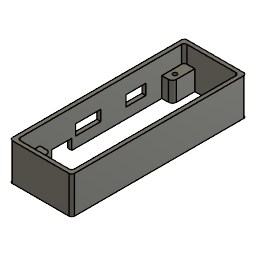
weather_station1 (Autodesk Fusion 360 design; units mm, degrees)
part number: 2026-01-11-18-10-58-376
Autodesk Fusion 360 part; units mm, degrees
sketch "Sketch11" plane through (0, 0, 0) normal (0, 1, 0) x (1, 0, 0)
  line L0 (0, 0) -> (47, 0)
  line L1 (47, 0) -> (47, -132)
  line L2 (47, -132) -> (0, -132)
  line L3 (0, -132) -> (0, 0)
  circle A0 centre (2, -2) radius 2
  circle A1 centre (45, -2) radius 2
  circle A2 centre (45, -130) radius 2
  circle A3 centre (2, -130) radius 2
  line L4 (3, -3) -> (44, -3)
  line L5 (44, -3) -> (44, -129)
  line L6 (44, -129) -> (3, -129)
  line L7 (3, -129) -> (3, -3)
  circle A4 centre (5, -5) radius 2
  circle A5 centre (42, -5) radius 2
  circle A6 centre (42, -127) radius 2
  circle A7 centre (5, -127) radius 2
  line L8 (3, -132) -> (6, -132)
  line L9 (6, -132) -> (6, -121)
  line L10 (6, -121) -> (3, -121)
  line L11 (3, -121) -> (3, -132)
  line L12 (44, -132) -> (41, -132)
  line L13 (41, -132) -> (41, -121)
  line L14 (41, -121) -> (44, -121)
  line L15 (44, -121) -> (44, -132)
  line L16 (3, 0) -> (6, 0)
  line L17 (6, 0) -> (6, -11)
  line L18 (6, -11) -> (3, -11)
  line L19 (3, -11) -> (3, 0)
  line L20 (44, 0) -> (41, 0)
  line L21 (41, 0) -> (41, -11)
  line L22 (41, -11) -> (44, -11)
  line L23 (44, -11) -> (44, 0)
  circle A8 centre (41, -11) radius 1
  circle A9 centre (6, -11) radius 1
  circle A10 centre (41, -121) radius 1
  circle A11 centre (6, -121) radius 1
  line L24 (3, -117) -> (9, -117)
  line L25 (9, -117) -> (9, -129)
  line L26 (9, -129) -> (3, -129)
  line L27 (3, -129) -> (3, -117)
  line L28 (44, -117) -> (38, -117)
  line L29 (38, -117) -> (38, -129)
  line L30 (38, -129) -> (44, -129)
  line L31 (44, -129) -> (44, -117)
  line L32 (44, -15) -> (38, -15)
  line L33 (38, -15) -> (38, -3)
  line L34 (38, -3) -> (44, -3)
  line L35 (44, -3) -> (44, -15)
  line L36 (3, -15) -> (9, -15)
  line L37 (9, -15) -> (9, -3)
  line L38 (9, -3) -> (3, -3)
  line L39 (3, -3) -> (3, -15)
  circle A12 centre (7, -13) radius 2
  circle A13 centre (40, -119) radius 2
  circle A14 centre (7, -119) radius 2
  circle A15 centre (40, -13) radius 2
  dimension "d82" = 47
  dimension "d83" = 132
  constraint horizontal L0
  constraint vertical L1
  constraint horizontal L2
  constraint vertical L3
  constraint coincident L0.start L3.end
  constraint tangent L0 A0
  constraint tangent L0 A1
  constraint tangent L1 A2
  constraint tangent L2 A3
  constraint horizontal L4
  constraint vertical L5
  constraint horizontal L6
  constraint vertical L7
  constraint tangent L4 A4
  constraint tangent L4 A5
  constraint tangent L5 A6
  constraint tangent L6 A7
  constraint horizontal L8
  constraint vertical L9
  constraint horizontal L10
  constraint vertical L11
  constraint coincident L2 L8.start
  constraint horizontal L12
  constraint vertical L13
  constraint horizontal L14
  constraint vertical L15
  constraint coincident L2 L12.start
  constraint horizontal L16
  constraint vertical L17
  constraint horizontal L18
  constraint vertical L19
  constraint coincident L0 L16.start
  constraint horizontal L20
  constraint vertical L21
  constraint horizontal L22
  constraint vertical L23
  constraint coincident L0 L20.start
  constraint coincident L21.end L22.start
  constraint coincident L17.end L18.start
  constraint coincident L13.end L14.start
  constraint coincident L9.end L10.start
  constraint horizontal L24
  constraint vertical L25
  constraint horizontal L26
  constraint vertical L27
  constraint coincident L6 L25.end
  constraint coincident L7 L24.start
  constraint horizontal L28
  constraint vertical L29
  constraint horizontal L30
  constraint vertical L31
  constraint coincident L5 L28.start
  constraint horizontal L32
  constraint vertical L33
  constraint horizontal L34
  constraint vertical L35
  constraint coincident L4 L33.end
  constraint coincident L5 L32.start
  constraint horizontal L36
  constraint vertical L37
  constraint horizontal L38
  constraint vertical L39
  constraint coincident L4 L37.end
  constraint coincident L7 L36.start
  constraint tangent L37 A12
  constraint tangent L28 A13
  constraint tangent L24 A14
  constraint tangent L32 A15
  measures "d82" distance of L0.start L0.end
  measures "d83" distance of L0.start L2.end
extrude "Extrude19" add sketch "Sketch11" along normal blind 3 contours L0 A0 L19 | L0 A0 L4 L16 L17 L19 L38 | L0 L4 L17 L21 L34 L38 | A0 L7 L19 L39 | A0 L4 L19 L38 | L0 A1 L4 L20 L21 L23 L34 | L3 A0 A3 L7 L11 L19 L27 L39 | A0 L4 L7 L19 L38 L39 | L0 A1 L23 | A0 L4 L7 A4 L19 L38 L39 | A3 L7 L11 L27 | A1 L5 L23 L35 | A1 L4 L23 L34 | A1 L4 L5 A5 L23 L34 L35 | A3 L6 L7 A7 L11 L26 L27 | A3 L6 L7 L11 L26 L27 | L2 A3 L11 | L1 A1 A2 L5 L15 L23 L31 L35 | A1 L4 L5 L23 L34 L35 | L2 A3 L6 L8 L9 L11 L26 | A3 L6 L11 L26 | A2 L5 L15 L31 | L2 L6 L9 L13 L26 L30 | A2 L5 L6 L15 L30 L31 | A2 L5 L6 A6 L15 L30 L31 | L2 A2 L15 | L2 A2 L6 L12 L13 L15 L30 | A2 L6 L15 L30 makes body 1
extrude "Extrude24" add 1 faces at (46, 3, 83) along direction (0, 1, 0) blind 25 on bodies 1 bodies 1
sketch "Sketch12" plane through (0, 0, 0) normal (-1, 0, 0) x (0, 0, 1)
  line L0 (2, 0) -> (130, 0)
  line L1 (130, 0) -> (130, 28)
  line L2 (130, 28) -> (2, 28)
  line L3 (2, 28) -> (2, 0)
  line L4 (132, 0) -> (121, 0)
  line L5 (121, 15) -> (132, 15)
  line L6 (132, 15) -> (132, 0)
  line L7 (121, 0) -> (101, 0)
  line L8 (121, 5) -> (121, 0)
  line L9 (121, 10) -> (121, 15)
  line L10 (121, 5) -> (121, 10)
  line L11 (69, 0) -> (121, 0)
  line L12 (121, 0) -> (121, 15)
  line L13 (0, 0) -> (11, 0)
  line L14 (11, 0) -> (11, 15)
  line L15 (11, 15) -> (0, 15)
  line L16 (0, 15) -> (0, 0)
  line L17 (11, 0) -> (31, 0)
  line L18 (31, 0) -> (31, 5)
  line L19 (31, 5) -> (11, 5)
  line L20 (11, 5) -> (11, 0)
  line L21 (31, 5) -> (11, 5)
  line L22 (11, 5) -> (11, 10)
  line L23 (11, 10) -> (31, 10)
  line L24 (31, 10) -> (31, 5)
  line L25 (31, 5) -> (41, 5)
  line L26 (41, 5) -> (41, 10)
  line L27 (41, 10) -> (31, 10)
  line L28 (31, 10) -> (31, 5)
  line L29 (41, 5) -> (41, 10)
  line L30 (41, 10) -> (41, 5)
  line L31 (41, 5) -> (62, 5)
  line L32 (62, 5) -> (62, 10)
  line L33 (62, 10) -> (41, 10)
  line L34 (41, 10) -> (41, 5)
  line L35 (62, 5) -> (80, 5)
  line L36 (80, 5) -> (80, 10)
  line L37 (80, 10) -> (62, 10)
  line L38 (62, 10) -> (62, 5)
  line L39 (121, 0) -> (101, 0)
  line L40 (101, 0) -> (101, 5)
  line L41 (101, 5) -> (121, 5)
  line L42 (121, 5) -> (121, 0)
  line L43 (101, 0) -> (91, 0)
  line L44 (91, 0) -> (91, 5)
  line L45 (91, 5) -> (101, 5)
  line L46 (101, 5) -> (101, 0)
  constraint horizontal L4
  constraint horizontal L5
  constraint vertical L6
  constraint horizontal L7
  constraint vertical L8
  constraint vertical L9
  constraint vertical L10
  constraint horizontal L11
  constraint vertical L12
  constraint coincident L0 L11.start
  constraint horizontal L13
  constraint vertical L14
  constraint horizontal L15
  constraint vertical L16
  constraint coincident L13.start L16.end
  constraint horizontal L17
  constraint vertical L18
  constraint horizontal L19
  constraint vertical L20
  constraint horizontal L21
  constraint vertical L22
  constraint horizontal L23
  constraint vertical L24
  constraint coincident L14 L22.end
  constraint horizontal L25
  constraint vertical L26
  constraint horizontal L27
  constraint vertical L28
  constraint vertical L29
  constraint vertical L30
  constraint horizontal L31
  constraint vertical L32
  constraint horizontal L33
  constraint vertical L34
  constraint horizontal L35
  constraint vertical L36
  constraint horizontal L37
  constraint vertical L38
  constraint horizontal L39
  constraint vertical L40
  constraint horizontal L41
  constraint vertical L42
  constraint horizontal L43
  constraint vertical L44
  constraint horizontal L45
  constraint vertical L46
extrude "Extrude25" cut sketch "Sketch12" against normal blind 3 contours L24 L25 L26 L27 L28 L29 L30 L34 | L0 L11 L40 L43 L44 L45 L46 | L32 L35 L36 L37 L38 bodies 1
sketch "Sketch13" plane through (0, 0, 0) normal (0, 1, 0) x (1, 0, 0)
  line L0 (70, 0) -> (118, 0)
  line L1 (118, 0) -> (118, -133)
  line L2 (118, -133) -> (70, -133)
  line L3 (70, -133) -> (70, 0)
  circle A0 centre (72, -2) radius 2
  circle A1 centre (116, -2) radius 2
  circle A2 centre (116, -131) radius 2
  circle A3 centre (72, -131) radius 2
  line L4 (67, 3) -> (121, 3)
  line L5 (121, 3) -> (121, -136)
  line L6 (121, -136) -> (67, -136)
  line L7 (67, -136) -> (67, 3)
  line L8 (118, 0) -> (126, 0)
  line L9 (126, 0) -> (126, 8)
  line L10 (126, 8) -> (118, 8)
  line L11 (118, 8) -> (118, 0)
  circle A4 centre (122, 4) radius 2
  line L12 (117, -1) -> (127, -1)
  line L13 (127, -1) -> (127, 9)
  line L14 (127, 9) -> (117, 9)
  line L15 (117, 9) -> (117, -1)
  circle A5 centre (66, 4) radius 2
  line L16 (70, 0) -> (62, 0)
  line L17 (62, 0) -> (62, 8)
  line L18 (62, 8) -> (70, 8)
  line L19 (70, 8) -> (70, 0)
  line L20 (71, -1) -> (61, -1)
  line L21 (61, -1) -> (61, 9)
  line L22 (61, 9) -> (71, 9)
  line L23 (71, 9) -> (71, -1)
  circle A6 centre (122, -137) radius 2
  line L24 (118, -133) -> (126, -133)
  line L25 (126, -133) -> (126, -141)
  line L26 (126, -141) -> (118, -141)
  line L27 (118, -141) -> (118, -133)
  line L28 (117, -132) -> (127, -132)
  line L29 (127, -132) -> (127, -142)
  line L30 (127, -142) -> (117, -142)
  line L31 (117, -142) -> (117, -132)
  line L32 (70, -133) -> (62, -133)
  line L33 (62, -133) -> (62, -141)
  line L34 (62, -141) -> (70, -141)
  line L35 (70, -141) -> (70, -133)
  line L36 (71, -132) -> (61, -132)
  line L37 (61, -132) -> (61, -142)
  line L38 (61, -142) -> (71, -142)
  line L39 (71, -142) -> (71, -132)
  circle A7 centre (66, -137) radius 2
  constraint horizontal L0
  constraint vertical L1
  constraint horizontal L2
  constraint vertical L3
  constraint tangent L0 A0
  constraint tangent L0 A1
  constraint tangent L2 A2
  constraint tangent L3 A3
  constraint horizontal L4
  constraint vertical L5
  constraint horizontal L6
  constraint vertical L7
  constraint horizontal L8
  constraint vertical L9
  constraint horizontal L10
  constraint vertical L11
  constraint horizontal L12
  constraint vertical L13
  constraint horizontal L14
  constraint vertical L15
  constraint horizontal L16
  constraint vertical L17
  constraint horizontal L18
  constraint vertical L19
  constraint horizontal L20
  constraint vertical L21
  constraint horizontal L22
  constraint vertical L23
  constraint horizontal L24
  constraint vertical L25
  constraint horizontal L26
  constraint vertical L27
  constraint horizontal L28
  constraint vertical L29
  constraint horizontal L30
  constraint vertical L31
  constraint horizontal L32
  constraint vertical L33
  constraint horizontal L34
  constraint vertical L35
  constraint horizontal L36
  constraint vertical L37
  constraint horizontal L38
  constraint vertical L39
copy_body "Body->Comp2" bodies 1 removing the originals makes body 2 in component "Component"
sketch "Sketch15" plane through (0, 0, 0) normal (0, 1, 0) x (1, 0, 0)
  line L0 (3, -112) -> (11, -112)
  line L1 (11, -112) -> (11, -129)
  line L2 (11, -129) -> (3, -129)
  line L3 (3, -129) -> (3, -112)
  line L4 (44, -112) -> (36, -112)
  line L5 (36, -112) -> (36, -129)
  line L6 (36, -129) -> (44, -129)
  line L7 (44, -129) -> (44, -112)
  line L8 (3, -20) -> (11, -20)
  line L9 (11, -20) -> (11, -3)
  line L10 (11, -3) -> (3, -3)
  line L11 (3, -3) -> (3, -20)
  line L12 (44, -20) -> (36, -20)
  line L13 (36, -20) -> (36, -3)
  line L14 (36, -3) -> (44, -3)
  line L15 (44, -3) -> (44, -20)
  circle A0 centre (7, -118) radius 1.5
  circle A1 centre (40, -118) radius 1.5
  circle A2 centre (7, -14) radius 1.5
  circle A3 centre (40, -14) radius 1.5
  dimension "d104" = 3
  dimension "d105" = 3
  dimension "d106" = 3
  dimension "d107" = 3
  constraint horizontal L0
  constraint vertical L1
  constraint horizontal L2
  constraint vertical L3
  constraint horizontal L4
  constraint vertical L5
  constraint horizontal L6
  constraint vertical L7
  constraint horizontal L8
  constraint vertical L9
  constraint horizontal L10
  constraint vertical L11
  constraint horizontal L12
  constraint vertical L13
  constraint horizontal L14
  constraint vertical L15
  measures "d104" diameter of A0
  measures "d105" diameter of A1
  measures "d106" diameter of A2
  measures "d107" diameter of A3
extrude "Extrude1" add sketch "Sketch15" along normal blind 15 bodies 2 in component "Component"
fillet "Fillet1" radius 3 1 edges at (11, 7.5, 20) on bodies 2 in component "Component"
fillet "Fillet2" radius 3 1 edges at (36, 7.5, 20) on bodies 2 in component "Component"
fillet "Fillet3" radius 3 1 edges at (11, 7.5, 112) on bodies 2 in component "Component"
fillet "Fillet4" radius 3 1 edges at (36, 7.5, 112) on bodies 2 in component "Component"
extrude "Extrude2" cut 1 faces at (1, 1.6667, 91) along direction (0, 0, -1) blind 3 on bodies 2 bodies 2 in component "Component"
extrude "Extrude3" cut 1 faces at (1, 1.6667, 101) along direction (0, 0, 1) blind 2 on bodies 2 bodies 2 in component "Component"
extrude "Extrude4" cut 1 faces at (1, 5, 93) along direction (0, 1, 0) blind 3 on bodies 2 bodies 2 in component "Component"
extrude "Extrude5" cut 1 faces at (1, 6.6667, 80) along direction (0, 0, 1) blind 5 on bodies 2 bodies 2 in component "Component"
extrude "Extrude6" add 1 faces at (1, 6.6667, 62) along direction (0, 0, 1) blind 4 on bodies 2 bodies 2 in component "Component"
extrude "Extrude7" cut 1 faces at (1, 10, 78.6667) along direction (0, 1, 0) blind 6 on bodies 2 bodies 2 in component "Component"
extrude "Extrude8" add 1 faces at (2, 5, 72.3333) along direction (0, 1, 0) blind 3 on bodies 2 bodies 2 in component "Component"
extrude "Extrude9" cut 1 faces at (1, 6.6667, 41) along direction (0, 0, 1) blind 6 on bodies 2 bodies 2 in component "Component"
extrude "Extrude10" add 1 faces at (1, 8.3333, 31) along direction (0, 0, 1) blind 1 on bodies 2 bodies 2 in component "Component"
extrude "Extrude11" cut 1 faces at (1, 10, 37) along direction (0, 1, 0) blind 6 on bodies 2 bodies 2 in component "Component"
extrude "Extrude12" add 1 faces at (1, 5, 37) along direction (0, 1, 0) blind 3 on bodies 2 bodies 2 in component "Component"
component "Component" placed x (1, 0, 0) y (0, 1, 0) z (0, 0, 1) at (0, 0, 0)
